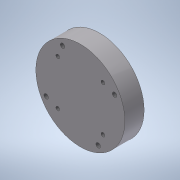
# Autodesk Inventor part: J010343
Saved by Autodesk Inventor 2020.3 (Build 243373000, 373)
## iProperties
RuleStatus: InUse
AfterDocSave0: file://Part Number Cleaner
Created: 2018-10-11
Material: ALUMINUM, 6061-T651
Vendor: HHMI: JRC - ID&F
Document SubType Name: Modeling
Designer: arnoldj
Density: 2.7 g/cm^3
Appearance: Metal-AL-6061 (Machined)
Description: VP AIR CYLINFER MOUNT
Project: COMMON
Part Number: J010343
LAB/DEPT: FLY FACILITY (SHARED RESOURCE)
REQUESTING SCIENTIST: COMMON
SURFACE ROUGHNESS: 64 Ra
DESIGN DEPARTMENT: HHMI: JRC - ID&F
SPECIAL FINISH: NONE
ALTERED ITEM PART NUMBER: N/A
ALTERED ITEM VENDOR: N/A
ALTERED ITEM DESCRIPTION: N/A
Author: arnoldj
Revision Number: -
Autodesk Inventor part; units mm, degrees
ref_plane "YZ Plane" through (0, 0, 0) normal (1, 0, 0) x (0, 1, 0)
ref_plane "XZ Plane" through (0, 0, 0) normal (0, 1, 0) x (-1, 0, 0)
ref_plane "XY Plane" through (0, 0, 0) normal (0, 0, 1) x (1, 0, 0)
sketch "Sketch1" plane through (0, 0, 0) normal (0, 0, 1) x (1, 0, 0)
  line L0 (0, 66.675) -> (0, -66.675) projected
  line L1 (-66.675, 0) -> (66.675, 0) projected
  circle A0 centre (0, 0) radius 47.625
  circle A1 centre (0, 0) radius 10.3188
  dimension "d0" = 20.6375
  dimension "d1" = 95.25
  constraints: 2 centre point, 2 coincident
  measures "d0" diameter of A1
  measures "d1" diameter of A0
extrude "Extrusion1" add sketch "Sketch1" along normal blind 20.574
sketch "Sketch2" plane through (0, 0, 0) normal (0, 0, -1) x (-1, 0, 0)
  line L0 (0, -66.675) -> (0, 66.675) projected
  line L1 (-66.675, 0) -> (66.675, 0) projected
  line L2 (-24.1554, -24.1554) -> (24.1554, -24.1554) construction
  line L3 (24.1554, -24.1554) -> (24.1554, 24.1554) construction
  line L4 (24.1554, 24.1554) -> (-24.1554, 24.1554) construction
  line L5 (-24.1554, 24.1554) -> (-24.1554, -24.1554) construction
  line L6 (-24.1554, -24.1554) -> (24.1554, 24.1554) construction
  line L7 (24.1554, -24.1554) -> (-24.1554, 24.1554) construction
  circle A0 centre (0, 0) radius 34.1609 construction
  dimension "d25" = 68.3218
  dimension "d22" = 48.3108
  constraints: 12 end point, 2 coincident, 2 midpoint, 2 parallel, 2 perpendicular, 1 horizontal, 3 other
  measures "d22" distance of L3.end L4.end
hole "Hole1" at (-24.1554, -24.1554, 0) direction (0, 0, 1) diameter 4.134 end through all thread size "M5x0.8" class "6H" standard "ANSI Metric M Profile"
sketch "Sketch3" plane through (0, 0, 20.574) normal (0, 0, 1) x (1, 0, 0)
  line L0 (0, 66.675) -> (0, -66.675) projected
  line L1 (-66.675, 0) -> (66.675, 0) projected
  circle A0 centre (0, 0) radius 41.275 construction
  line L2 (0, 0) -> (-36.6114, -19.0587) construction
  point P0 (-24.1554, -24.1554)
  point P1 (-24.1554, -24.1554)
  dimension "d23" = 82.55
  dimension "d24" = 62.5
  constraints: 3 coincident, 2 end point, 3 other
  measures "d24" angle of L2 L0
hole "Hole2" at (-36.6114, -19.0587, 20.574) direction (0, 0, -1) diameter 4.917 end through all thread size "M6x1" class "6H" standard "ANSI Metric M Profile"
pattern_circular "Circular Pattern1" count 4 over 360 about axis through (0, 0, -10) along (0, 0, 1) of "Hole1", "Hole2"
body "Solid1"
